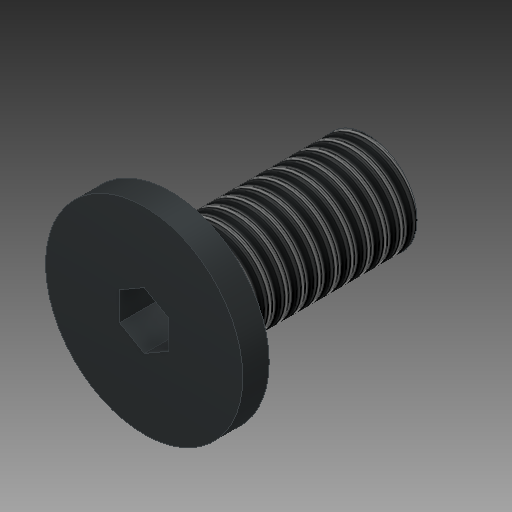
# Autodesk Inventor part: M3ネジ　スリムヘッド　6
Saved by Autodesk Inventor 2017.3 (Build 213256000, 256)
## iProperties
Part Number: M3ネジ　スリムヘッド　6
Material: 鉄 灰色
Document SubType Name: Modeling
Designer: 原知也
Density: 7.15 g/cm^3
Appearance: 鉄 灰色
Mass: 0.449646 g
Surface Area: 1.33893 cm^2
Volume: 0.0628876 cm^3
Author: 原知也
Autodesk Inventor part; units mm, degrees
ref_plane "YZ Plane" through (0, 0, 0) normal (1, 0, 0) x (0, 1, 0)
ref_plane "XZ Plane" through (0, 0, 0) normal (0, 1, 0) x (-1, 0, 0)
ref_plane "XY Plane" through (0, 0, 0) normal (0, 0, 1) x (1, 0, 0)
sketch "スケッチ1" plane through (0, 0, 0) normal (0, 0, 1) x (1, 0, 0)
  circle A0 centre (0, 0) radius 1.5
  dimension "d0" = 3
  constraints: 1 centre point, 1 coincident
  measures "d0" diameter of A0
extrude "押し出し1" add sketch "スケッチ1" along normal blind 6
sketch "スケッチ2" plane through (0, 0, 6) normal (0, 0, 1) x (1, 0, 0)
  circle A0 centre (0, 0) radius 3
  dimension "d3" = 6
  constraints: 1 centre point, 1 coincident
  measures "d3" diameter of A0
extrude "押し出し2" add sketch "スケッチ2" along normal blind 0.8
sketch "スケッチ3" plane through (0, 0, 6.8) normal (0, 0, 1) x (1, 0, 0)
  line L0 (0, 0.866) -> (0.75, 0.433)
  line L1 (0.75, 0.433) -> (0.75, -0.433)
  line L2 (0.75, -0.433) -> (0, -0.866)
  line L3 (0, -0.866) -> (-0.75, -0.433)
  line L4 (-0.75, -0.433) -> (-0.75, 0.433)
  line L5 (-0.75, 0.433) -> (0, 0.866)
  point P0 (0, 0)
  point P1 (0, 0)
  dimension "d7" = 1.5
  constraints: 12 end point, 1 coincident, 13 other
  measures "d7" distance between parallel lines of L1 L4
extrude "押し出し3" cut sketch "スケッチ3" against normal blind 1.1
thread "ねじ1" size "M3x0.5" class "6g" standard "ANSI Metric M Profile" full length
